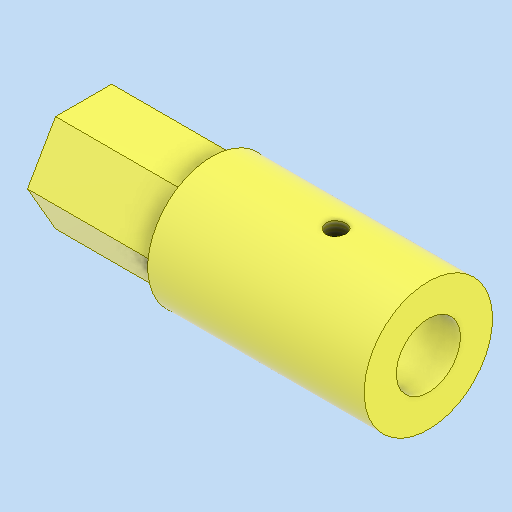
# Autodesk Inventor part: переходная втулка
Saved by Autodesk Inventor 2025 (Build 290162000, 162)
## iProperties
Created: 2025-02-17
Part Number: переходная втулка
Material: Типовые
Document SubType Name: Modeling
Designer: volko
Density: 1 g/cm^3
Appearance: Гладкий — желтый
Mass: 6.42234 g
Surface Area: 30.4849 cm^2
Volume: 6.42234 cm^3
Author: volko
Autodesk Inventor part; units mm, degrees
ref_plane "YZ Plane" through (0, 0, 0) normal (1, 0, 0) x (0, 1, 0)
ref_plane "XY Plane" through (0, 0, 0) normal (0, 0, 1) x (1, 0, 0)
sketch "Эскиз1" plane through (0, 0, 0) normal (1, 0, 0) x (0, 1, 0)
  line L0 (6.0622, 3.5) -> (6.0622, -3.5)
  line L1 (6.0622, -3.5) -> (0, -7)
  line L2 (0, -7) -> (-6.0622, -3.5)
  line L3 (-6.0622, -3.5) -> (-6.0622, 3.5)
  line L4 (-6.0622, 3.5) -> (0, 7)
  line L5 (0, 7) -> (6.0622, 3.5)
  circle A0 centre (0, 0) radius 7 construction
  dimension "d0" = 14
  constraints: 12 end point, 2 coincident, 1 vertical, 16 other
extrude "Выдавливание1" add sketch "Эскиз1" along normal blind 25
sketch "Эскиз2" plane through (25, 0, 0) normal (1, 0, 0) x (0, 0, -1)
  circle A0 centre (0, 0) radius 8
  circle A1 centre (0, 0) radius 4
  dimension "d3" = 16
  dimension "d6" = 8
  constraints: 2 centre point, 2 coincident
  measures "d3" diameter of A0
  measures "d6" diameter of A1
extrude "Выдавливание2" add sketch "Эскиз2" along normal blind 18 and the other way blind 9
ref_plane "РабПлоскость1" through (0, 9, 0) normal (0, 1, 0) x (-1, 0, 0)
sketch "Эскиз3" plane through (0, 9, 0) normal (0, 1, 0) x (-1, 0, 0)
  line L0 (-43, 8) -> (-43, -8) projected
  point P0 (0, 0)
  point P1 (-31.5, 0)
  dimension "d16" = 11.5
  measures "d16" distance from line of L0 point (-31.5, 0)
hole "Отверстие1" at (31.5, 9, 0) direction (0, -1, 0) diameter 2.459 end through all thread size "M3x0.5" class "6H" standard "ISO Metric profile"
sketch "Эскиз4" plane through (0, 0, 0) normal (-1, 0, 0) x (0, 0, 1)
  point P0 (0, 0)
  point P1 (0, 0)
  constraints: 1 coincident
hole "Отверстие2" at (0, 0, 0) direction (1, 0, 0) diameter 3.242 depth 11.8 tip angle 118 thread size "M4x0.7" class "6H" standard "ISO Metric profile"
